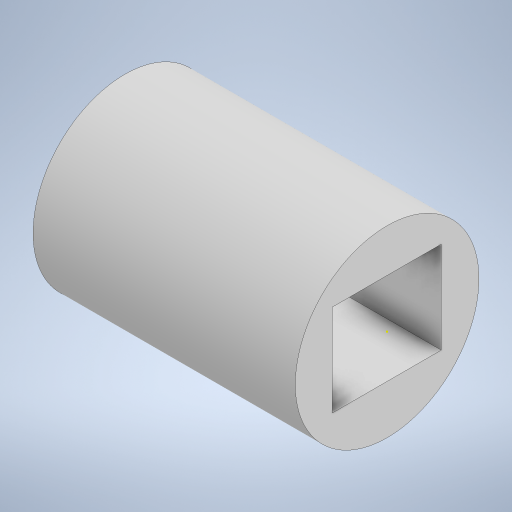
# Autodesk Inventor part: Wkp 01.03
Saved by Autodesk Inventor 2023 (Build 270158000, 158)
## iProperties
Created: 2023-03-01
Part Number: Wkp 01.03
Material: Generic
Document SubType Name: Modeling
Designer: accam
Density: 1 g/cm^3
Appearance: Default
Author: accam
Autodesk Inventor part; units mm, degrees
ref_plane "YZ Plane" through (0, 0, 0) normal (1, 0, 0) x (0, 1, 0)
ref_plane "XZ Plane" through (0, 0, 0) normal (0, 1, 0) x (-1, 0, 0)
ref_plane "XY Plane" through (0, 0, 0) normal (0, 0, 1) x (1, 0, 0)
sketch "Sketch1" plane through (0, 0, 0) normal (1, 0, 0) x (0, 1, 0)
  circle A0 centre (0, 0) radius 3.5
  dimension "d7" = 7
  constraints: 1 centre point, 1 coincident
  measures "d7" diameter of A0
extrude "Extrusion1" add sketch "Sketch1" along normal blind 10
sketch "Sketch2" plane through (0, 0, 0) normal (-1, 0, 0) x (0, 0, 1)
  line L0 (2.0913, 1.859) -> (-2.064, 1.859)
  line L1 (-2.064, 1.859) -> (-2.064, -1.6403)
  line L2 (-2.064, -1.6403) -> (2.0913, -1.6403)
  line L3 (2.0913, -1.6403) -> (2.0913, 1.859)
  point P0 (0, 0)
  constraints: 8 end point, 2 parallel, 1 horizontal, 1 perpendicular
sketch "Sketch4" plane through (10, 0, 0) normal (1, 0, 0) x (0, 0, -1)
  point P0 (0, 0)
extrude "Extrusion2" cut sketch "Sketch2" against normal blind 16.25
body "Solid1"
